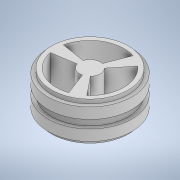
# Autodesk Inventor part: Dubbele wiel
Saved by Autodesk Inventor 2022 (Build 260153000, 153)
## iProperties
Created: 2022-11-03
Part Number: Dubbele wiel
Material: Generic
Document SubType Name: Modeling
Designer: Kilian De Ruyck
Density: 1 g/cm^3
Appearance: Default
Author: Kilian De Ruyck
Autodesk Inventor part; units mm, degrees
ref_plane "YZ Plane" through (0, 0, 0) normal (1, 0, 0) x (0, 1, 0)
ref_plane "XZ Plane" through (0, 0, 0) normal (0, 1, 0) x (-1, 0, 0)
ref_plane "XY Plane" through (0, 0, 0) normal (0, 0, 1) x (1, 0, 0)
sketch "Sketch1" plane through (0, 0, 0) normal (0, 1, 0) x (-1, 0, 0)
  circle A0 centre (0, 0) radius 14.25
  dimension "d0" = 28.5
  constraints: 1 centre point, 1 coincident
  measures "d0" diameter of A0
extrude "Extrusion1" add sketch "Sketch1" along normal blind 3.7
sketch "Sketch2" plane through (0, 3.7, 0) normal (0, 1, 0) x (1, 0, 0)
  circle A0 centre (0, 0) radius 13
  dimension "d3" = 26
  constraints: 1 centre point, 1 coincident
  measures "d3" diameter of A0
extrude "Extrusion2" add sketch "Sketch2" along normal blind 1.4
sketch "Sketch3" plane through (0, 0, 0) normal (0, -1, 0) x (1, 0, 0)
  circle A0 centre (0, 0) radius 13
  dimension "d6" = 26
  constraints: 1 centre point, 1 coincident
  measures "d6" diameter of A0
extrude "Extrusion3" add sketch "Sketch3" along normal blind 1.4
sketch "Sketch4" plane through (0, 5.1, 0) normal (0, 1, 0) x (1, 0, 0)
  circle A0 centre (0, 0) radius 13
  dimension "d9" = 26
  constraints: 1 centre point, 1 coincident
  measures "d9" diameter of A0
extrude "Extrusion4" add sketch "Sketch4" along normal blind 1.4
sketch "Sketch5" plane through (0, 6.5, 0) normal (0, 1, 0) x (1, 0, 0)
  circle A0 centre (0, 0) radius 14.25
  constraints: 1 centre point, 1 coincident
extrude "Extrusion5" add sketch "Sketch5" along normal blind 3.7
sketch "Sketch6" plane through (0, 10.2, 0) normal (0, 1, 0) x (1, 0, 0)
  circle A0 centre (0, 0) radius 13
  dimension "d14" = 26
  constraints: 1 centre point, 1 coincident
  measures "d14" diameter of A0
extrude "Extrusion6" add sketch "Sketch6" along normal blind 1.4
sketch "Sketch7" plane through (0, -1.4, 0) normal (0, -1, 0) x (1, 0, 0)
  circle A0 centre (0, 0) radius 3.5
  circle A1 centre (0, 0) radius 11.5
  line L0 (0, 0) -> (-11.5, 0)
  line L1 (0, 0) -> (11.5, 0) construction
  line L2 (0, 0) -> (5.75, -9.9593)
  line L3 (0, 0) -> (11.5, 0) construction
  line L4 (1.75, -3.0311) -> (0.8214, -3.4022)
  line L5 (5.75, -9.9593) -> (3.7007, -10.8883)
  line L6 (5.75, -9.9593) -> (7.5792, -8.6491)
  line L7 (3.7007, -10.8883) -> (0.8214, -3.4022)
  line L8 (1.75, -3.0311) -> (2.5357, -2.4125)
  line L9 (2.5357, -2.4125) -> (7.5792, -8.6491)
  line L10 (0, 0) -> (-11.5, 0)
  line L11 (0, 0) -> (5.75, 9.9593)
  line L12 (0, 0) -> (11.5, 0) construction
  line L13 (0.8214, 3.4022) -> (3.7007, 10.8883)
  line L14 (1.75, 3.0311) -> (0.8214, 3.4022)
  line L15 (1.75, 3.0311) -> (2.5357, 2.4125)
  line L16 (7.5792, 8.6491) -> (2.5357, 2.4125)
  line L17 (5.75, 9.9593) -> (3.7007, 10.8883)
  line L18 (5.75, 9.9593) -> (7.5792, 8.6491)
  line L19 (-3.3571, -0.9897) -> (-11.2799, -2.2392)
  line L20 (-3.5, 0) -> (-3.3571, -0.9897)
  line L21 (-3.5, 0) -> (-3.3571, 0.9897)
  line L22 (-11.2799, 2.2392) -> (-3.3571, 0.9897)
  line L23 (-11.5, 0) -> (-11.2799, -2.2392)
  line L24 (-11.5, 0) -> (-11.2799, 2.2392)
  dimension "d17" = 7
  dimension "d20" = 60
  dimension "d21" = 1
  dimension "d23" = 2.25
  dimension "d24" = 2.25
  dimension "d27" = 1
  dimension "d28" = 60
  dimension "d31" = 360
  constraints: 50 end point, 8 point on circle, 4 horizontal, 2 centre point, 2 coincident, 2 equal length, 1 collinear, 1 point on line, 37 other
  measures "d17" diameter of A0
  measures "d20" angle of L2 L3
  measures "d21" distance of L4.start L4.end
  measures "d23" distance of L2.end L5.end
  measures "d24" distance of L2.end L6.end
  measures "d27" distance of L4.start L8.end
  measures "d28" angle of L12 L11
extrude "Extrusion7" cut sketch "Sketch7" against normal blind 20.15 contours A0 L16 A1 L9 | A0 L22 A1 L13 | L7 A1 L19 A0
sketch "Sketch8" plane through (0, -1.4, 0) normal (0, -1, 0) x (1, 0, 0)
  circle A0 centre (0, 0) radius 1.625
  line L0 (0, 0) -> (-0.8125, -1.4073)
  line L1 (0, 0) -> (1.625, 0) construction
  line L2 (-0.8125, -1.4073) -> (0.5625, 0.9743)
  line L3 (0.5625, 0.9743) -> (1.578, 0.388)
  line L4 (0.5625, 0.9743) -> (-0.453, 1.5606)
  dimension "d35" = 3.25
  dimension "d36" = 120
  dimension "d37" = 2.75
  constraints: 10 end point, 3 point on circle, 2 point on line, 1 centre point, 1 coincident, 1 equal length, 1 horizontal
  measures "d35" diameter of A0
  measures "d36" angle of L0 L1
  measures "d37" distance of L0.end L2.end
extrude "Extrusion8" cut sketch "Sketch8" against normal blind 8 contours A0 L0 L2 L3 | A0 L4 L2 L0
sketch "Sketch9" plane through (0, -1.4, 0) normal (0, -1, 0) x (1, 0, 0)
  line L0 (0, 0) -> (-2.083, -3.6079)
  line L1 (0, 0) -> (4.166, 0) construction
  arc A0 (-3.3571, -0.9897) -> (0.8214, -3.4022) centre (0, 0) ccw projected
  line L2 (-2.8281, -2.8985) -> (-0.9783, -3.6945)
  line L3 (0, 0) -> (-0.654, 0.3671)
  line L4 (-0.654, 0.3671) -> (0.654, -0.3671)
  line L5 (0.654, -0.3671) -> (-1.5061, -4.1613)
  line L6 (-0.654, 0.3671) -> (-2.9167, -3.5519)
  line L7 (-0.654, 0.3671) -> (3.8713, 0.3671) construction
  point P0 (-2.5969, -2.998)
  point P1 (-1.1888, -3.6039)
  dimension "d40" = 120
  dimension "d45" = 0.75
  dimension "d46" = 1.5
  dimension "d47" = 120
  constraints: 16 end point, 2 equal length, 2 horizontal, 1 point on line
  measures "d40" angle of L0 L1
  measures "d45" distance of L3.start L3.end
  measures "d46" distance of L3.end L4.end
  measures "d47" angle of L6 L7
extrude "Extrusion9" cut sketch "Sketch9" against normal blind 8
body "Solid1"
